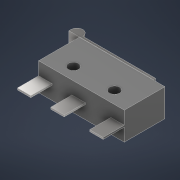
# Autodesk Inventor part: LimitSwitch_V1
Saved by Autodesk Inventor 2022.2 (Build 262287000, 287)
## iProperties
Created: 2023-05-21
Part Number: LimitSwitch_V1
Material: Acetal Resin, Black
Document SubType Name: Modeling
Designer: jaege
Density: 1.425 g/cm^3
Appearance: Smooth - Black
Author: jaege
Autodesk Inventor part; units mm, degrees
ref_plane "YZ Plane" through (0, 0, 0) normal (1, 0, 0) x (0, 1, 0)
ref_plane "XZ Plane" through (0, 0, 0) normal (0, 1, 0) x (-1, 0, 0)
ref_plane "XY Plane" through (0, 0, 0) normal (0, 0, 1) x (1, 0, 0)
sketch "Sketch1" plane through (0, 0, 0) normal (0, 1, 0) x (-1, 0, 0)
  line L0 (-9.9, 4.7) -> (9.9, 4.7)
  line L1 (9.9, 4.7) -> (9.9, -4.7)
  line L2 (9.9, -4.7) -> (-9.9, -4.7)
  line L3 (-9.9, -4.7) -> (-9.9, 4.7)
  line L4 (-9.9, 4.7) -> (9.9, -4.7) construction
  line L5 (9.9, 4.7) -> (-9.9, -4.7) construction
  line L6 (12.5, -5.4) -> (-6.5, -5.4)
  line L7 (-6.5, -5.4) -> (-6.5, -4.9)
  line L8 (-6.5, -4.9) -> (12.5, -4.9)
  line L9 (12.5, -4.9) -> (12.5, -5.4)
  line L10 (-6.5, -5.4) -> (-7, -5.4)
  line L11 (-7, -5.4) -> (-7, -4.7)
  line L12 (-7, -4.7) -> (-6.5, -4.7)
  line L13 (-6.5, -4.7) -> (-6.5, -5.4)
  arc A0 (12.5, -5.4) -> (9.8, -5.4) centre (11.15, -5.4) ccw construction
  arc A1 (9.8, -5.4) -> (12.5, -5.4) centre (11.15, -5.4) ccw
  point P0 (0, 0)
  point P1 (-7, -5.05)
  dimension "d0" = 19.8
  dimension "d1" = 9.4
  dimension "d2" = 0.5
  dimension "d3" = 0.5
  dimension "d4" = 0.7
  dimension "d5" = 19
  dimension "d6" = 2.7
  dimension "d7" = 2.9
  constraints: 28 end point, 6 parallel, 4 point on circle, 3 horizontal, 3 midpoint, 3 perpendicular, 3 point on line, 2 centre point
  measures "d0" distance of L1.end L2.end
  measures "d1" distance of L0.end L1.end
  measures "d2" distance of L6.end L10.end
  measures "d3" distance of L8.end L6.start
  measures "d4" distance of L10.end L11.end
  measures "d5" distance of L6.start L6.end
  measures "d6" diameter of A0
  measures "d7" distance from line of L3 point (-7, -5.05)
extrude "Extrusion1" add sketch "Sketch1" along normal blind 6.4
sketch "Sketch3" plane through (-9.9, 0, 4.7) normal (0, 0, 1) x (1, 0, 0)
  line L0 (0, 3) -> (3.1, 3)
  line L1 (3.1, 3) -> (3.1, 3.4)
  line L2 (3.1, 3.4) -> (0, 3.4)
  line L3 (0, 3.4) -> (0, 3)
  line L4 (7.7, 3) -> (10.8, 3)
  line L5 (10.8, 3) -> (10.8, 3.4)
  line L6 (10.8, 3.4) -> (7.7, 3.4)
  line L7 (7.7, 3.4) -> (7.7, 3)
  line L8 (16.7, 3.4) -> (19.8, 3.4)
  line L9 (19.8, 3.4) -> (19.8, 3)
  line L10 (19.8, 3) -> (16.7, 3)
  line L11 (16.7, 3) -> (16.7, 3.4)
  line L12 (-2.6, 6.4) -> (16.4, 6.4) projected
  line L13 (19.8, 0) -> (16.9, 0) projected
  line L14 (-2.6, 6.4) -> (19.8, 0) construction
  line L15 (19.8, 0) -> (19.8, 6.4) projected
  line L16 (0, 0) -> (0, 6.4) projected
  point P0 (9.9, 0)
  point P1 (0, 3.2)
  point P2 (8.6, 3.2)
  point P3 (19.8, 3.2)
  dimension "d10" = 3.1
  dimension "d11" = 0.4
  dimension "d12" = 9
  constraints: 26 end point, 6 parallel, 4 collinear, 3 horizontal, 3 midpoint, 3 perpendicular, 3 point on line, 1 horizontal alignment, 1 vertical alignment
  measures "d10" distance of L1.end L2.end
  measures "d11" distance of L2.end L0.start
  measures "d12" distance from line of L15 L5.end
extrude "Extrusion2" add sketch "Sketch3" along normal blind 4.9
sketch "Sketch4" plane through (0, 6.4, 0) normal (0, 1, 0) x (1, 0, 0)
  line L0 (-12.5, 5.4) -> (-12.5, 4.9) projected
  line L1 (-12.5, 4.9) -> (6.5, 4.9) projected
  line L2 (6.5, 4.9) -> (6.5, 4.7) projected
  line L3 (6.5, 4.7) -> (-9.9, 4.7) projected
  line L4 (-9.9, 4.7) -> (-9.9, -4.7) projected
  line L5 (-9.9, -4.7) -> (9.9, -4.7) projected
  line L6 (9.9, -4.7) -> (9.9, 4.7) projected
  line L7 (9.9, 4.7) -> (7, 4.7) projected
  line L8 (7, 4.7) -> (7, 5.4) projected
  line L9 (7, 5.4) -> (-9.8, 5.4) projected
  arc A0 (-9.8, 5.4) -> (-12.5, 5.4) centre (-11.15, 5.4) ccw projected
  line L10 (6.5, 4.9) -> (6.5, 4.7) projected
  line L11 (6.5, 4.7) -> (7, 4.7)
  point P0 (0, 0)
  constraints: 2 end point, 1 perpendicular
extrude "Extrusion3" cut sketch "Sketch4" against normal blind 0.1 contours A0 L9 L8 L11 L2 L1 L0
sketch "Sketch5" plane through (0, 0, 0) normal (0, -1, 0) x (1, 0, 0)
  line L0 (-12.5, -5.4) -> (-12.5, -4.9) projected
  arc A0 (-12.5, -5.4) -> (-9.8, -5.4) centre (-11.15, -5.4) ccw projected
  line L1 (7, -5.4) -> (-9.8, -5.4) projected
  line L2 (7, -4.7) -> (7, -5.4) projected
  line L3 (9.9, -4.7) -> (7, -4.7) projected
  line L4 (9.9, 4.7) -> (9.9, -4.7) projected
  line L5 (-9.9, 4.7) -> (9.9, 4.7) projected
  line L6 (-9.9, -4.7) -> (-9.9, 4.7) projected
  line L7 (6.5, -4.7) -> (-9.9, -4.7) projected
  line L8 (6.5, -4.9) -> (6.5, -4.7) projected
  line L9 (-12.5, -4.9) -> (6.5, -4.9) projected
  line L10 (7, -4.7) -> (6.5, -4.7) projected
  line L11 (7, -4.7) -> (6.5, -4.7)
  point P0 (0, 0)
  constraints: 2 end point, 1 collinear
extrude "Extrusion4" cut sketch "Sketch5" against normal blind 0.1 contours L0 L9 L8 L10 L2 L1 A0
sketch "Sketch6" plane through (0, 6.4, 0) normal (0, 1, 0) x (1, 0, 0)
  circle A0 centre (-4.75, -1.8) radius 1.175
  circle A1 centre (4.75, -1.8) radius 1.175
  line L0 (-4.75, -1.8) -> (4.75, -1.8) construction
  line L1 (-9.9, -4.7) -> (9.9, -4.7) projected
  point P0 (0, 0)
  point P1 (0, -1.8)
  dimension "d19" = 2.35
  dimension "d20" = 9.5
  dimension "d21" = 2.9
  constraints: 2 centre point, 2 end point, 1 equal radius, 1 horizontal, 1 horizontal alignment, 1 midpoint, 1 vertical alignment
  measures "d19" diameter of A0
  measures "d20" distance of L0.end L0.start
  measures "d21" distance from line of L1 L0.start
extrude "Extrusion5" cut sketch "Sketch6" against normal up to surface (6.4 mm away)
body "Solid1"
